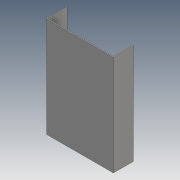
# Autodesk Inventor part: Part1
Saved by Autodesk Inventor 2016 SP1 (Build 200210100, 210)
## iProperties
Created: 2017-02-23
Part Number: Part1
Material: Generic
Document SubType Name: Modeling
Designer: Fraser Muir
Density: 1 g/cm^3
Appearance: Default
Author: Fraser Muir
Autodesk Inventor part; units mm, degrees
note: some values were not read from the file. Chosen so that the rebuilt part matches the saved one: sketch regions of "Extrusion2".
ref_plane "YZ Plane" through (0, 0, 0) normal (1, 0, 0) x (0, 1, 0)
ref_plane "XZ Plane" through (0, 0, 0) normal (0, 1, 0) x (-1, 0, 0)
ref_plane "XY Plane" through (0, 0, 0) normal (0, 0, 1) x (1, 0, 0)
sketch "Sketch1" plane through (0, 0, 0) normal (0, 0, 1) x (1, 0, 0)
  line L0 (0, 0) -> (10000, 0)
  line L1 (10000, 0) -> (10000, -3000)
  line L2 (10000, -3000) -> (0, -3000)
  line L3 (0, -3000) -> (0, 0)
  dimension "d0" = 10000
  dimension "d1" = 3000
  constraints: 8 end point, 2 parallel, 1 horizontal, 1 perpendicular
  measures "d0" distance of L1.end L2.end
  measures "d1" distance of L0.end L1.end
extrude "Extrusion1" add sketch "Sketch1" along normal blind 15000
sketch "Sketch2" plane through (0, 0, 0) normal (0, 1, 0) x (1, 0, 0)
  line L0 (0, 0) -> (10000, 0) projected
  line L1 (0, 0) -> (0, -15000) projected
  line L2 (10000, -15000) -> (0, -15000) projected
  line L3 (10000, 0) -> (10000, -15000) projected
  line L4 (9900, -14900) -> (100, -14900)
  line L5 (100, -14900) -> (100, -100)
  line L6 (100, -100) -> (9900, -100)
  line L7 (9900, -100) -> (9900, -14900)
  line L8 (9900, -14900) -> (9900, -15000)
  line L9 (10000, 0) -> (10000, -15000) projected
  line L10 (9900, -15000) -> (10000, -15000)
  line L11 (100, -14900) -> (100, -15000)
  line L12 (10000, -15000) -> (0, -15000) projected
  line L13 (100, -15000) -> (0, -15000)
  line L14 (9900, -8277.7517) -> (100, -8277.7517)
  line L15 (100, -8277.7517) -> (100, -8377.7517)
  line L16 (100, -8377.7517) -> (9900, -8377.7517)
  line L17 (9900, -8377.7517) -> (9900, -8277.7517)
  line L18 (5000, -8377.7517) -> (5000, -8277.7517)
  line L19 (7000, -8277.7517) -> (3000, -8277.7517)
  line L20 (3000, -8277.7517) -> (3000, -8377.7517)
  line L21 (3000, -8377.7517) -> (7000, -8377.7517)
  line L22 (7000, -8377.7517) -> (7000, -8277.7517)
  line L23 (7000, -8277.7517) -> (3000, -8377.7517) construction
  line L24 (3000, -8277.7517) -> (7000, -8377.7517) construction
  line L25 (100, -8277.7517) -> (600, -8277.7517)
  line L26 (600, -8277.7517) -> (600, -8377.7517)
  line L27 (600, -8377.7517) -> (100, -8377.7517)
  line L28 (100, -8377.7517) -> (100, -8277.7517)
  line L29 (9900, -8277.7517) -> (9400, -8277.7517)
  line L30 (9400, -8277.7517) -> (9400, -8377.7517)
  line L31 (9400, -8377.7517) -> (9900, -8377.7517)
  line L32 (9900, -8377.7517) -> (9900, -8277.7517)
  point P0 (5000, -8327.7517)
  dimension "d4" = 100
  dimension "d5" = 100
  dimension "d6" = 4000
  dimension "d7" = 100
  dimension "d14" = 500
  dimension "d15" = 500
  constraints: 54 end point, 8 parallel, 6 perpendicular, 6 point on line, 5 horizontal, 5 midpoint, 1 collinear, 3 other
  measures "d4" distance between parallel lines of L3 L7
  measures "d5" distance of L15.end L14.end
  measures "d6" distance of L21.end L20.end
  measures "d7" distance of L20.end L19.end
  measures "d14" distance of L26.end L27.end
  measures "d15" distance of L31.end L30.end
extrude "Extrusion2" cut sketch "Sketch2" against normal blind 2900 contours L11 L4 L8 L2 | L5 L16 L7 L4 | L5 L6 L7 L14
extrude "Extrusion3" cut sketch "Sketch2" against normal blind 2900 contours L5 L14 L26 L16 | L16 L30 L14 L7 | L26 L14 L20 L16 | L16 L22 L14 L30 | L20 L14 L18 L16 | L16 L18 L14 L22
extrude "Extrusion4" add sketch "Sketch2" against normal blind 2900 contours L5 L14 L26 L16 | L16 L30 L14 L7 | L20 L14 L18 L16 | L16 L18 L14 L22
sketch "Sketch3" plane through (0, 0, 0) normal (0, 0, -1) x (-1, 0, 0)
  line L0 (-100, 0) -> (-9900, 0) projected
  line L1 (-100, 0) -> (-100, -2900) projected
  line L2 (-9900, -2900) -> (-100, -2900) projected
  line L3 (-9900, 0) -> (-9900, -2900) projected
  line L4 (-150, -50) -> (-150, -2850)
  line L5 (-9850, -2900) -> (-9850, -50)
  line L6 (-9900, -2900) -> (-100, -2900) projected
  line L7 (-150, -2900) -> (-150, -50)
  line L8 (-9850, -50) -> (-7910, -50)
  line L9 (-7910, -50) -> (-7910, -2900)
  line L10 (-7910, -2900) -> (-9850, -2900)
  line L11 (-9850, -2900) -> (-9850, -50)
  line L12 (-7860, -50) -> (-7860, -2900)
  line L13 (-9850, -50) -> (-7910, -50)
  line L14 (-7910, -50) -> (-7910, -2900)
  line L15 (-7910, -2900) -> (-9850, -2900)
  line L16 (-9850, -2900) -> (-9850, -50)
  line L17 (-9850, -50) -> (-7910, -50)
  line L18 (-7910, -50) -> (-7910, -2900)
  line L19 (-7910, -2900) -> (-9850, -2900)
  line L20 (-9850, -2900) -> (-9850, -50)
  line L21 (-7910, -2900) -> (-7910, -50)
  line L22 (-7910, -50) -> (-5970, -50)
  line L23 (-5970, -50) -> (-5970, -2900)
  line L24 (-5970, -2900) -> (-7910, -2900)
  line L25 (-5920, -50) -> (-5920, -2900)
  line L26 (-5970, -2900) -> (-5970, -50)
  line L27 (-5970, -50) -> (-4030, -50)
  line L28 (-4030, -50) -> (-4030, -2900)
  line L29 (-4030, -2900) -> (-5970, -2900)
  line L30 (-3980, -50) -> (-3980, -2900)
  line L31 (-4030, -2900) -> (-4030, -50)
  line L32 (-4030, -50) -> (-2090, -50)
  line L33 (-2090, -50) -> (-2090, -2900)
  line L34 (-2090, -2900) -> (-4030, -2900)
  line L35 (-2040, -50) -> (-2040, -2900)
  line L36 (-2090, -2900) -> (-2090, -50)
  line L37 (-2090, -50) -> (-150, -50)
  line L38 (-150, -50) -> (-150, -2900)
  line L39 (-150, -2900) -> (-2090, -2900)
  line L40 (-100, -50) -> (-100, -2900)
  line L41 (-9850, -50) -> (-7910, -50)
  line L42 (-7910, -50) -> (-7910, -2900)
  line L43 (-7910, -2900) -> (-9850, -2900)
  line L44 (-9850, -2900) -> (-9850, -50)
  line L45 (-7860, -50) -> (-5970, -50)
  line L46 (-5970, -50) -> (-5970, -2900)
  line L47 (-5970, -2900) -> (-7860, -2900)
  line L48 (-7860, -2900) -> (-7860, -50)
  line L49 (-5920, -50) -> (-4030, -50)
  line L50 (-4030, -50) -> (-4030, -2900)
  line L51 (-4030, -2900) -> (-5920, -2900)
  line L52 (-5920, -2900) -> (-5920, -50)
  line L53 (-3980, -50) -> (-2090, -50)
  line L54 (-2090, -50) -> (-2090, -2900)
  line L55 (-2090, -2900) -> (-3980, -2900)
  line L56 (-3980, -2900) -> (-3980, -50)
  line L57 (-2040, -2900) -> (-150, -2900)
  line L58 (-150, -2900) -> (-150, -50)
  line L59 (-150, -50) -> (-2040, -50)
  line L60 (-2040, -50) -> (-2040, -2900)
  line L61 (-100, -2900) -> (-100, 0) projected
  line L62 (-9900, 0) -> (-9900, -2900) projected
  line L63 (-100, 0) -> (-9900, 0)
  line L64 (-9900, 0) -> (-9900, -2900)
  line L65 (-9900, -2900) -> (-100, -2900)
  line L66 (-100, -2900) -> (-100, 0)
  line L67 (-7910, -50) -> (-7860, -50)
  line L68 (-7860, -50) -> (-7860, -2900)
  line L69 (-7860, -2900) -> (-7910, -2900)
  line L70 (-7910, -2900) -> (-7910, -50)
  line L71 (-5970, -2900) -> (-5920, -2900)
  line L72 (-5920, -2900) -> (-5920, -50)
  line L73 (-5920, -50) -> (-5970, -50)
  line L74 (-5970, -50) -> (-5970, -2900)
  line L75 (-4030, -50) -> (-3980, -50)
  line L76 (-3980, -50) -> (-3980, -2900)
  line L77 (-3980, -2900) -> (-4030, -2900)
  line L78 (-4030, -2900) -> (-4030, -50)
  line L79 (-2090, -2900) -> (-2040, -2900)
  line L80 (-2040, -2900) -> (-2040, -50)
  line L81 (-2040, -50) -> (-2090, -50)
  line L82 (-2090, -50) -> (-2090, -2900)
  point P0 (0, 0)
  dimension "d17" = 9700
  dimension "d18" = 1940
  dimension "d19" = 50
  dimension "d22" = 1940
  constraints: 152 end point, 26 parallel, 14 horizontal, 14 perpendicular, 2 collinear, 2 point on line, 1 coincident, 51 other
  measures "d17" distance of L5.end L4.start
  measures "d18" distance of L9.end L10.end
  measures "d19" distance between parallel lines of L12 L9
  measures "d22" distance of L5.start L21.start
extrude "Extrusion5" cut sketch "Sketch3" against normal blind 25 contours L5 L8 L9 L2 | L2 L35 L37 L4 L7 | L12 L22 L23 L2 | L2 L30 L32 L33 | L25 L27 L28 L2
sketch "Sketch4" plane through (100, 0, 100) normal (0, 0, 1) x (1, 0, 0)
  line L0 (9750, -2900) -> (9750, -50) projected
  line L1 (7810, -2900) -> (9750, -2900) projected
  line L2 (7810, -50) -> (7810, -2900) projected
  line L3 (9750, -50) -> (7810, -50) projected
  line L4 (5870, -2900) -> (7760, -2900) projected
  line L5 (5870, -50) -> (5870, -2900) projected
  line L6 (7760, -50) -> (5870, -50) projected
  line L7 (7760, -2900) -> (7760, -50) projected
  line L8 (5820, -2900) -> (5820, -50) projected
  line L9 (3930, -2900) -> (5820, -2900) projected
  line L10 (3930, -50) -> (3930, -2900) projected
  line L11 (5820, -50) -> (3930, -50) projected
  line L12 (1990, -2900) -> (3880, -2900) projected
  line L13 (1990, -50) -> (1990, -2900) projected
  line L14 (3880, -50) -> (1990, -50) projected
  line L15 (3880, -2900) -> (3880, -50) projected
  line L16 (1940, -2900) -> (1940, -50) projected
  line L17 (50, -2900) -> (1940, -2900) projected
  line L18 (50, -50) -> (50, -2900) projected
  line L19 (1940, -50) -> (50, -50) projected
  point P0 (-100, 0)
extrude "Extrusion6" cut sketch "Sketch4" against normal blind 25
sketch "Sketch5" plane through (3000, 0, 8377.7517) normal (0, 0, 1) x (1, 0, 0)
  point P0 (-3000, 0)
body "Solid1"
